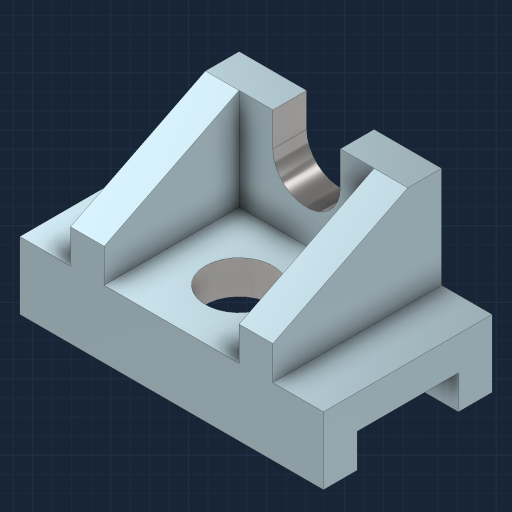
# Autodesk Inventor part: s14-12
Saved by Autodesk Inventor 2024 (Build 280153000, 153)
## iProperties
Created: 2026-04-09
Part Number: s14-12
Material: Generic
Document SubType Name: Modeling
Designer: DuctopwH
Density: 1 g/cm^3
Appearance: Default
Author: DuctopwH
Autodesk Inventor part; units mm, degrees
ref_plane "YZ Plane" through (0, 0, 0) normal (1, 0, 0) x (0, 1, 0)
ref_plane "XZ Plane" through (0, 0, 0) normal (0, 1, 0) x (-1, 0, 0)
ref_plane "XY Plane" through (0, 0, 0) normal (0, 0, 1) x (1, 0, 0)
sketch "Sketch1" plane through (0, 0, 0) normal (1, 0, 0) x (0, 1, 0)
  line L0 (-5, 25) -> (5, 25)
  line L1 (5, 25) -> (5, -25)
  line L2 (5, -25) -> (-5, -25)
  line L3 (-5, -25) -> (-5, 25)
  line L4 (-5, 25) -> (5, -25) construction
  line L5 (5, 25) -> (-5, -25) construction
  line L6 (-5, -25) -> (-15, -25)
  line L7 (-15, -25) -> (-15, -15)
  line L8 (-15, -15) -> (-5, -15)
  line L9 (-5, -15) -> (-5, -25)
  line L10 (5, 0) -> (-34.0233, 0) construction
  line L11 (-5, 25) -> (-15, 25)
  line L12 (-15, 25) -> (-15, 15)
  line L13 (-15, 15) -> (-5, 15)
  point P0 (0, 0)
  point P1 (-15, -20)
  dimension "d0" = 50
  dimension "d1" = 10
  dimension "d2" = 10
  dimension "d3" = 20
  constraints: 28 end point, 4 midpoint, 4 parallel, 3 horizontal, 3 symmetric about line, 2 perpendicular
  measures "d0" distance of L0.end L1.end
  measures "d1" distance from line of L3 point (-15, -20)
  measures "d2" distance of L6.end L7.end
  measures "d3" distance between parallel lines of L1 L7
extrude "Extrusion1" add sketch "Sketch1" along normal mid plane 90
sketch "Sketch2" plane through (45, 5, -25) normal (0, 0, -1) x (-1, 0, 0)
  line L0 (0, 0) -> (90, 0) projected
  line L1 (0, -20) -> (0, 0) projected
  line L2 (90, -20) -> (0, -20) projected
  line L3 (90, 0) -> (90, -20) projected
  line L4 (15, 0) -> (75, 0)
  line L5 (75, 0) -> (75, 30)
  line L6 (75, 30) -> (15, 30)
  line L7 (15, 30) -> (15, 0)
  point P0 (45, -5)
  point P1 (45, 30)
  dimension "d6" = 50
  dimension "d7" = 60
  constraints: 8 end point, 2 parallel, 1 horizontal, 1 midpoint, 1 perpendicular, 1 point on line, 1 vertical alignment
  measures "d6" distance between parallel lines of L6 L2
  measures "d7" distance of L5.end L6.end
extrude "Extrusion2" add sketch "Sketch2" against normal blind 10 contours L7 L6 L5 L0
sketch "Sketch3" plane through (-30, 5, -25) normal (-1, 0, 0) x (0, 0, 1)
  line L0 (0, 30) -> (10, 30) projected
  line L1 (0, 0) -> (50, 0) projected
  line L2 (10, 30) -> (50, 10)
  line L3 (50, 0) -> (50, -20) projected
  line L4 (50, 0) -> (50, 10)
  line L5 (40, -20) -> (50, -20) projected
  line L6 (0, 0) -> (0, 30) projected
  point P0 (25, -5)
  dimension "d28" = 30
  constraints: 4 end point, 1 vertical
  measures "d28" distance from line of L5 L2.end
extrude "Extrusion4" add sketch "Sketch3" against normal blind 10
mirror "Mirror1" about plane through (0, 0, 0) normal (1, 0, 0) of "Extrusion4"
sketch "Sketch4" plane through (45, 5, -15) normal (0, 0, 1) x (1, 0, 0)
  circle A0 centre (-45, 20) radius 10
  line L0 (-55, 20) -> (-55, 30)
  line L1 (-15, 30) -> (-75, 30) projected
  line L2 (-45, 30) -> (-45, 0) construction
  line L3 (-15, 0) -> (-75, 0) projected
  line L4 (-35, 20) -> (-35, 30)
  point P0 (-45, -5)
  point P1 (-25, 30)
  point P2 (-65, 30)
  point P3 (-25, 0)
  point P4 (-65, 0)
  point P5 (-45, 10)
  point P6 (-35, 20)
  dimension "d16" = 20
  dimension "d17" = 20
  constraints: 6 end point, 3 point on line, 2 midpoint, 2 point on circle, 2 symmetric about line, 1 centre point, 1 tangent, 1 vertical
  measures "d16" diameter of A0
  measures "d17" distance from line of L1 A0.end
extrude "Extrusion3" cut sketch "Sketch4" against normal through all
sketch "Sketch5" plane through (-20, 5, 25) normal (0, 1, 0) x (1, 0, 0)
  line L0 (40, 40) -> (30, 40) projected
  line L1 (0, 0) -> (40, 0) projected
  point P0 (20, 20)
  point P1 (50, 40)
  point P2 (20, 0)
  dimension "d20" = 20
  constraints: 1 midpoint, 1 vertical alignment
  measures "d20" distance from line of L0 point (20, 20)
hole "Hole1" at (0, 5, 5) direction (0, -1, 0) diameter 20 end through all
body "Solid1"
